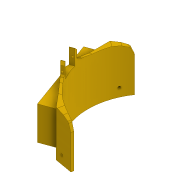
# Autodesk Inventor part: Delta Robot Mirrord Siding Piece
Saved by Autodesk Inventor 2020 (Build 240168000, 168)
## iProperties
Created: 2021-04-12
Part Number: Delta Robot Mirrord Siding Piece
Material: Generic
Document SubType Name: Modeling
Designer: Coy
Density: 1 g/cm^3
Appearance: Gold
Author: Coy
Autodesk Inventor part; units mm, degrees
ref_plane "YZ Plane" through (0, 0, 0) normal (1, 0, 0) x (0, 1, 0)
ref_plane "XZ Plane" through (0, 0, 0) normal (0, 1, 0) x (-1, 0, 0)
ref_plane "XY Plane" through (0, 0, 0) normal (0, 0, 1) x (1, 0, 0)
sketch "Sketch1" plane through (0, 0, 0) normal (0, 1, 0) x (-1, 0, 0)
  line L0 (68.675, -46.4884) -> (71.2969, -48.6885)
  line L1 (86.05, -31.1064) -> (71.2969, -48.6885)
  line L2 (86.05, 31.5329) -> (86.05, -31.1064)
  line L3 (45.7862, 79.5174) -> (86.05, 31.5329)
  line L4 (22.3355, 83.6524) -> (45.7862, 79.5174)
  line L5 (22.3355, 83.6524) -> (21.7555, 80.3631)
  arc A0 (68.675, -46.4884) -> (21.7555, 80.3631) centre (0, 0.2133) ccw
  constraints: 12 end point, 2 point on circle, 1 centre point
extrude "Extrusion1" add sketch "Sketch1" along normal blind 60
sketch "Sketch2" plane through (-86.05, 0, -31.1064) normal (-0.7660444, 0, -0.6427876) x (-0.6427876, 0, 0.7660444)
  circle A0 centre (-8.4518, 11) radius 1.625
  line L0 (-22.9518, 0) -> (0, 0) projected
  line L1 (-22.9518, 0) -> (-22.9518, 60) projected
  point P0 (-31.483, 0)
  dimension "d2" = 3.25
  dimension "d3" = 11
  dimension "d4" = 14.5
  constraints: 1 centre point
  measures "d2" diameter of A0
  measures "d3" distance from line of L0 A0.centre
  measures "d4" distance from line of L1 A0.centre
extrude "Extrusion2" cut sketch "Sketch2" against normal up to next
sketch "Sketch3" plane through (-22.3355, 0, 83.6524) normal (-0.1736482, 0, 0.9848078) x (0.9848078, 0, 0.1736482)
  circle A0 centre (-14.5, 11) radius 1.625
  line L0 (-23.8125, 0) -> (0, 0) projected
  line L1 (0, 0) -> (0, 60) projected
  point P0 (7.4701, 0)
  dimension "d7" = 3.25
  dimension "d8" = 11
  dimension "d9" = 14.5
  constraints: 1 centre point
  measures "d7" diameter of A0
  measures "d8" distance from line of L0 A0.centre
  measures "d9" distance from line of L1 A0.centre
extrude "Extrusion3" cut sketch "Sketch3" against normal up to next
sketch "Sketch4" plane through (0, 60, 0) normal (0, 1, 0) x (1, 0, 0)
  line L0 (-81.5111, -16.1268) -> (-86.05, -17.7788)
  line L1 (-86.05, -17.7788) -> (-86.05, -31.5329)
  line L2 (-86.05, -31.5329) -> (-80.5261, -38.116)
  line L3 (-80.5261, -38.116) -> (-74.9097, -36.0718)
  arc A0 (-81.5111, -16.1268) -> (-74.9097, -36.0718) centre (0, -0.2133) ccw
  line L4 (-22.3355, -83.6524) -> (-21.7555, -80.3631) projected
  arc A1 (-68.675, 46.4884) -> (-21.7555, -80.3631) centre (0, -0.2133) ccw projected
  line L5 (-68.675, 46.4884) -> (-71.2969, 48.6885) projected
  line L6 (-71.2969, 48.6885) -> (-86.05, 31.1064) projected
  line L7 (-86.05, 31.1064) -> (-86.05, -31.5329) projected
  line L8 (-86.05, -31.5329) -> (-45.7862, -79.5174) projected
  line L9 (-45.7862, -79.5174) -> (-22.3355, -83.6524) projected
  line L10 (-86.642, -17.3643) -> (-81.0601, -15.3327)
  arc A2 (-81.0601, -15.3327) -> (-74.0916, -36.404) centre (0, -0.2133) ccw construction
  line L11 (-74.0916, -36.404) -> (-80.7131, -38.8141)
  line L12 (-80.7131, -38.8141) -> (-86.642, -31.7484) construction
  line L13 (-86.642, -31.7484) -> (-86.642, -17.3643) construction
  line L14 (-78.2508, -10.5574) -> (-90.1684, -14.8951)
  line L15 (-90.1684, -14.8951) -> (-90.1684, -33.0319) construction
  line L16 (-90.1684, -33.0319) -> (-81.8274, -42.9724) construction
  line L17 (-81.8274, -42.9724) -> (-69.1104, -38.3438)
  arc A3 (-78.2508, -10.5574) -> (-69.1104, -38.3438) centre (0, -0.2133) ccw construction
  line L18 (-86.05, -31.5329) -> (-45.7862, -79.5174) construction
  line L19 (-86.05, -31.5329) -> (-90.1684, -33.0319) construction
  line L20 (-72.6702, -40.4171) -> (-77.2091, -42.0691)
  line L21 (-77.2091, -42.0691) -> (-86.05, -31.5329)
  line L22 (-86.05, -31.5329) -> (-86.05, -22.9392)
  line L23 (-86.05, -22.9392) -> (-80.4336, -20.895)
  arc A4 (-80.4336, -20.895) -> (-72.6702, -40.4171) centre (0, -0.2133) ccw
  line L24 (-77.3961, -42.7671) -> (-71.8142, -40.7355)
  arc A5 (-80.0204, -20.1147) -> (-71.8142, -40.7355) centre (0, -0.2133) ccw construction
  line L25 (-80.0204, -20.1147) -> (-86.642, -22.5247)
  line L26 (-86.642, -22.5247) -> (-86.642, -31.7484) construction
  line L27 (-86.642, -31.7484) -> (-77.3961, -42.7671) construction
  line L28 (-66.5927, -42.5878) -> (-78.5103, -46.9255)
  line L29 (-78.5103, -46.9255) -> (-90.1684, -33.0319) construction
  line L30 (-90.1684, -33.0319) -> (-90.1684, -20.0555) construction
  line L31 (-90.1684, -20.0555) -> (-77.4515, -15.4269)
  arc A6 (-77.4515, -15.4269) -> (-66.5927, -42.5878) centre (0, -0.2133) ccw construction
  point P0 (0, 0)
  point P1 (0, 0)
  point P2 (-77.7089, -41.4734)
  point P3 (-73.0252, -39.7687)
  point P4 (-74.6509, -36.6076)
  point P5 (-80.1212, -38.5986)
  point P6 (-82.2096, -11.9983)
  point P7 (-86.05, -13.3961)
  point P8 (-86.05, -17.1489)
  point P9 (-81.6239, -15.5379)
  point P10 (-74.3919, -45.4265)
  point P11 (-70.5515, -44.0287)
  point P12 (-72.378, -40.9407)
  point P13 (-76.8041, -42.5517)
  point P14 (-86.05, -22.3093)
  point P15 (-80.5797, -20.3183)
  point P16 (-81.3662, -16.8517)
  point P17 (-86.05, -18.5565)
  dimension "d12" = 0.5919
  dimension "d13" = 3.5265
  constraints: 50 end point, 13 symmetric about line, 12 point on circle, 6 centre point, 11 other
  measures "d12" distance between parallel lines of L0 L10
  measures "d13" distance between parallel lines of L10 L14
extrude "Extrusion4" add sketch "Sketch4" along normal blind 20 contours A0 L25 L1 L31 | A1 L28 L8 L24
sketch "Sketch5" plane through (-70.5515, 60, 44.0287) normal (0.3420201, 0, 0.9396926) x (0.9396926, 0, -0.3420201)
  line L0 (-4.0869, 0) -> (-4.0869, 20) construction
  line L1 (-4.0869, 10) -> (0, 10) construction
  line L2 (0, 0) -> (0, 20) construction
  circle A0 centre (-2.0434, 10) radius 1.25
  point P0 (81.3554, -60)
  dimension "d18" = 2.5
  constraints: 3 midpoint, 2 end point, 1 centre point, 1 horizontal
  measures "d18" diameter of A0
extrude "Extrusion5" cut sketch "Sketch5" against normal up to next
sketch "Sketch6" plane through (-81.3662, 60, 16.8517) normal (-0.3420201, 0, -0.9396926) x (-0.9396926, 0, 0.3420201)
  line L0 (4.9844, 0) -> (4.9844, 20) construction
  line L1 (4.9844, 10) -> (0, 10) construction
  line L2 (0, 0) -> (0, 20) construction
  circle A0 centre (2.4922, 10) radius 1.25
  point P0 (-82.2229, -60)
  dimension "d21" = 2.5
  constraints: 3 midpoint, 2 end point, 1 centre point, 1 horizontal
  measures "d21" diameter of A0
extrude "Extrusion6" cut sketch "Sketch6" against normal up to next
chamfer "Chamfer1" distance 3 angle 45 2 edges at (-83.7081, 80, 17.7041) (-72.4717, 80, 44.7276)
chamfer "Chamfer2" distance 7 angle 45 2 edges at (-72.4717, 60, 44.7276) (-83.7081, 60, 17.7041)
chamfer "Chamfer3" distance 7 angle 45 2 edges at (-68.04, 60, 50.5639) (-84.2717, 60, 10.46)
chamfer "Chamfer4" distance 7 angle 45 2 edges at (-63.2913, 60, 56.2847) (-84.5335, 60, 3.106)
chamfer "Chamfer5" distance 10 angle 45 2 edges at (-22.0455, 60, 82.0077) (-69.9859, 60, -47.5884)
chamfer "Chamfer6" distance 7 angle 45 2 edges at (-31.7611, 60, 79.5197) (-75.788, 60, -39.4028)
chamfer "Chamfer7" distance 5 angle 45 2 edges at (-38.4957, 60, 77.4021) (-79.5549, 60, -33.4258)
chamfer "Chamfer8" distance 5 angle 45 2 edges at (-22.0455, 50, 82.0077) (-69.9859, 50, -47.5884)
ref_plane "Work Plane2" through (-107.6629, 60, -23.2399) normal (0.9396926, 0, -0.3420201) x (0.3420201, 0, 0.9396926)
ref_plane "Work Plane1" through (-86.05, 60, -31.1064) normal (0.9396926, 0, -0.3420201) x (0.3420201, 0, 0.9396926)
sketch "Sketch7" plane through (-107.6629, 60, -23.2399) normal (0.9396926, 0, -0.3420201) x (0.3420201, 0, 0.9396926)
  line L0 (0, 60) -> (0, 0) construction
  line L1 (117.7233, 60) -> (117.7233, 0) construction
  line L2 (58.8617, 60) -> (117.7233, 60) construction
  line L3 (0, 60) -> (58.8617, 60) construction
  line L4 (0, 0) -> (25.6678, 0) construction
  line L5 (96.9047, 0) -> (117.7233, 0) construction
  line L6 (109.7233, 8) -> (8, 8)
  line L7 (8, 8) -> (8, 52)
  line L8 (8, 52) -> (58.8617, 52)
  line L9 (58.8617, 52) -> (109.7233, 52)
  line L10 (109.7233, 52) -> (109.7233, 8)
  point P0 (58.6613, 60)
  dimension "d49" = 8
  constraints: 10 end point, 3 other
  measures "d49" distance between parallel lines of L0 L7
extrude "Extrusion7" add sketch "Sketch7" along normal up to next
body "Solid1"
